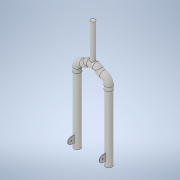
# Autodesk Inventor part: 前桿2
Saved by Autodesk Inventor 2020 (Build 240168000, 168)
## iProperties
Created: 2021-03-29
Part Number: 前桿2
Material: 一般
Document SubType Name: Modeling
Designer: cadlab
Density: 1 g/cm^3
Appearance: 預設
Author: cadlab
Autodesk Inventor part; units mm, degrees
sketch "草圖1" plane through (0, 0, 0) normal (0, 0, 1) x (1, 0, 0)
  line L0 (0, 0) -> (0, 12)
  line L1 (125, -79.4987) -> (125, -80)
  arc A0 (45, -10) -> (25, 0) centre (25, -25) ccw
  arc A1 (45, -10) -> (80, -29.7494) centre (85, 20) ccw
  arc A2 (125, -79.4987) -> (80, -29.7494) centre (75, -79.4987) ccw
  line L2 (125, -80) -> (125, -110)
  line L3 (25, 0) -> (0, 0)
  line L4 (-125, -79.4987) -> (-125, -80)
  arc A3 (-25, 0) -> (-45, -10) centre (-25, -25) ccw
  arc A4 (-80, -29.7494) -> (-45, -10) centre (-85, 20) ccw
  arc A5 (-80, -29.7494) -> (-125, -79.4987) centre (-75, -79.4987) ccw
  line L5 (-125, -80) -> (-125, -110)
  line L6 (-25, 0) -> (0, 0)
  line L7 (125, -110) -> (125, -470)
  line L8 (-125, -110) -> (-125, -470)
  dimension "d8" = 50
  dimension "d9" = 50
  dimension "d10" = 30
  dimension "d11" = 110
  dimension "d12" = 25
  dimension "d13" = 250
  dimension "d29" = 360
  constraints: 18 end point, 12 point on circle, 10 symmetric about line, 6 centre point, 3 tangent, 2 vertical, 1 horizontal, 3 other
  measures "d8" radius of A1
  measures "d9" radius of A2
  measures "d10" distance of L1.end L2.end
  measures "d11" vertical distance of L2.end L0.start
  measures "d12" radius of A0
  measures "d13" distance of L2.end L5.end
  measures "d29" distance of L2.end L7.end
ref_plane "工作平面1" through (0, 0, 0) normal (0, 1, 0) x (-1, 0, 0)
sketch "草圖2" plane through (0, 0, 0) normal (0, 1, 0) x (-1, 0, 0)
  circle A0 centre (0, 0) radius 17.5
  dimension "d14" = 35
  constraints: 1 centre point, 1 coincident
  measures "d14" diameter of A0
extrude "擠出1" add sketch "草圖2" along normal blind 300
ref_plane "工作平面2" through (-125, -110, 0) normal (0, -1, 0) x (1, 0, 0)
sketch "草圖3" plane through (-125, -110, 0) normal (0, -1, 0) x (1, 0, 0)
  circle A0 centre (0, 0) radius 27.5
  point P0 (125, 0)
  dimension "d17" = 55
  constraints: 1 centre point
  measures "d17" diameter of A0
sweep "掃掠1" add profiles "草圖3" path "草圖1" path curves L5 L4 A5 A4 A3 L6 L3 A0 A1 A2 L1 L2
ref_plane "工作平面6" through (-125, -470, 0) normal (0, -1, 0) x (1, 0, 0)
sketch "草圖15" plane through (125, -110, 0) normal (0, -1, 0) x (1, 0, 0)
  circle A0 centre (0, 0) radius 25
  circle A1 centre (-250, 0) radius 25
  circle A2 centre (-250, 0) radius 27.5 projected
  circle A3 centre (0, 0) radius 27.5 projected
  point P0 (-125, 0)
  dimension "d92" = 50
  dimension "d93" = 50
  constraints: 2 centre point, 2 concentric
  measures "d92" diameter of A0
  measures "d93" diameter of A1
extrude "擠出11" add sketch "草圖15" along normal blind 525 contours A0 | A1
ref_plane "工作平面11" through (125, 0, 0) normal (1, 0, 0) x (0, 1, 0)
ref_plane "工作平面8" through (125, -470, 0) normal (0, -1, 0) x (1, 0, 0)
ref_plane "工作平面9" through (125, 0, 0) normal (1, 0, 0) x (0, 1, 0)
sketch "草圖11" plane through (125, 0, 0) normal (1, 0, 0) x (0, 1, 0)
  arc A0 (-540.1241, 52.4876) -> (-589.8759, 52.4876) centre (-565, 50) ccw
  line L0 (-534.8753, 0) -> (-540.1241, 52.4876)
  line L1 (-589.8759, 52.4876) -> (-595.1247, 0)
  circle A1 centre (-565, 50) radius 5
  line L2 (-534.8753, 0) -> (-595.1247, 0)
  line L3 (-635, 25) -> (-635, -25) projected
  line L4 (-635, 0) -> (-565, 0)
  point P0 (0, 0)
  dimension "d99" = 70
  dimension "d100" = 25
  dimension "d101" = 50
  dimension "d102" = 10
  constraints: 8 end point, 2 centre point, 2 horizontal, 2 point on circle, 2 tangent, 1 coincident, 1 midpoint
  measures "d99" distance from line of L3 A0.centre
  measures "d100" radius of A0
  measures "d101" distance from line of L2 A0.centre
  measures "d102" diameter of A1
extrude "擠出8" add sketch "草圖11" along normal mid plane 5
mirror "鏡射1" about plane through (0, 0, 0) normal (1, 0, 0) of "擠出8"
